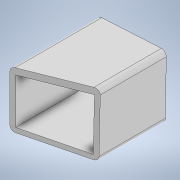
# Autodesk Inventor part: handle_top_final
Saved by Autodesk Inventor 2021 (Build 250183000, 183)
## iProperties
Created: 2021-09-13
Part Number: handle_top_final
Material: Generisch
Document SubType Name: Modeling
Designer: Alexander Claas
Density: 1 g/cm^3
Appearance: Vorgabe
Author: Alexander Claas
Autodesk Inventor part; units mm, degrees
ref_plane "YZ Plane" through (0, 0, 0) normal (1, 0, 0) x (0, 1, 0)
ref_plane "XZ Plane" through (0, 0, 0) normal (0, 1, 0) x (-1, 0, 0)
ref_plane "XY Plane" through (0, 0, 0) normal (0, 0, 1) x (1, 0, 0)
sketch "Skizze1" plane through (0, 0, 0) normal (0, 0, 1) x (1, 0, 0)
  line L0 (0, 0) -> (-40.8899, -4.2977)
  line L1 (-40.8899, -4.2977) -> (-40.8899, -33.7977)
  line L2 (-40.8899, -33.7977) -> (-0.5899, -33.7977)
  line L3 (-0.5899, -33.7977) -> (0, 0)
  line L4 (-43.8899, -0.591) -> (3.0763, 4.3454)
  line L5 (-43.8899, -36.7977) -> (-43.8899, -0.591)
  line L6 (-43.8899, -36.7977) -> (2.3582, -36.7977)
  line L7 (2.3582, -36.7977) -> (3.0763, 4.3454)
  dimension "d1" = 29.5
  dimension "d2" = 40.3
  dimension "d6" = 90
  dimension "d9" = 91
  dimension "d12" = 96
  dimension "d13" = 41.1152
  dimension "d14" = 33.8028
  dimension "d22" = 4
  dimension "d23" = 3
  dimension "d24" = 3
  dimension "d25" = 3
  constraints: 16 end point, 4 parallel, 1 vertical
  measures "d1" distance of L0.end L1.end
  measures "d2" distance of L1.end L2.end
  measures "d6" angle of L2 L1
  measures "d9" angle of L2 L3
  measures "d12" angle of L1 L0
  measures "d13" distance of L0.start L0.end
  measures "d14" distance of L2.end L0.start
  measures "d22" distance between parallel lines of L0 L4
  measures "d23" distance between parallel lines of L5 L1
  measures "d24" distance between parallel lines of L6 L2
  measures "d25" distance between parallel lines of L7 L3
extrude "Extrusion1" add sketch "Skizze1" along normal blind 57
sketch "Skizze3" plane through (-43.8899, -36.7977, 0) normal (0, -1, 0) x (1, 0, 0)
  line L0 (0, 0) -> (46.2481, 0) construction
  line L1 (46.2481, 0) -> (46.2481, 57) construction
  line L2 (0, 57) -> (46.2481, 57) construction
  line L3 (0, 0) -> (0, 57) projected
  line L4 (0, 0) -> (46.2481, 0)
  line L5 (0, 57) -> (46.2481, 57) projected
  line L6 (0, 57) -> (46.9662, 45.29)
  line L7 (46.2481, 0) -> (46.2481, 57) projected
  line L8 (46.2481, 0) -> (46.9662, 0) projected
  line L9 (46.2481, 0) -> (46.9662, 0)
  line L10 (46.9662, 0) -> (46.9662, 2.4614)
  line L11 (46.9662, 2.4614) -> (0, 0)
  line L12 (46.9662, 0) -> (46.9662, 57) projected
  line L13 (46.9662, 45.29) -> (46.9662, 57)
  line L14 (46.9662, 57) -> (46.9662, 57)
  line L15 (0, 57) -> (46.9662, 57)
  point P0 (43.8899, 0)
  dimension "d27" = 76
  dimension "d30" = 87
  constraints: 16 end point, 2 perpendicular, 1 horizontal, 1 vertical
  measures "d27" angle of L6 L3
  measures "d30" angle of L3 L11
extrude "Extrusion3" cut sketch "Skizze3" against normal blind 57 contours L11 L7 L4 | L5 L7 L6 | L7 L11 L10 L8 | L15 L12 L6 L7
fillet "Rundung1" radius 3 4 edges at (-43.8899, -36.7977, 28.5) (-43.8899, -0.591, 28.5) (2.3582, -36.7977, 23.9464) (3.0763, 4.3454, 23.8757)
equation "\"d24\" = d23"
equation "\"d25\" = d24"
